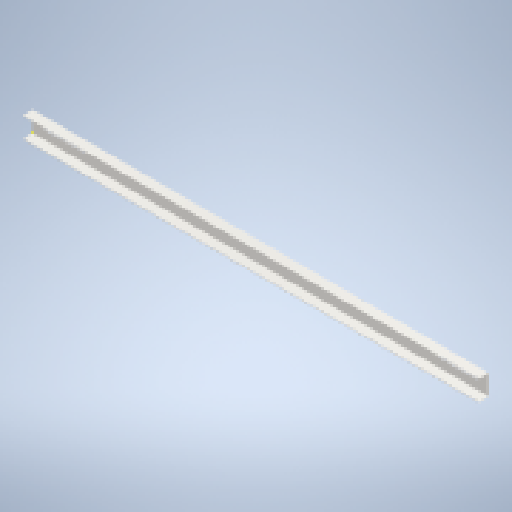
# Autodesk Inventor part: ThanhKe
Saved by Autodesk Inventor 2023 (Build 270158000, 158)
## iProperties
Created: 2025-03-24
Part Number: ThanhKe
Material: Generic
Document SubType Name: Modeling
Designer: huyqu
Density: 1 g/cm^3
Appearance: Default
Author: huyqu
Autodesk Inventor part; units mm, degrees
ref_plane "YZ Plane" through (0, 0, 0) normal (1, 0, 0) x (0, 1, 0)
ref_plane "XZ Plane" through (0, 0, 0) normal (0, 1, 0) x (-1, 0, 0)
ref_plane "XY Plane" through (0, 0, 0) normal (0, 0, 1) x (1, 0, 0)
sketch "Sketch1" plane through (0, 0, 0) normal (0, 0, 1) x (1, 0, 0)
  line L0 (0, 0) -> (2200, 0)
  line L1 (0, 0) -> (0, -3)
  line L2 (0, -3) -> (2200, -3)
  line L3 (2200, -3) -> (2200, 0)
  dimension "d0" = 2200
  dimension "d1" = 3
  dimension "d2" = 2200
  constraints: 8 end point, 2 horizontal, 1 vertical
  measures "d0" distance of L0.start L0.end
  measures "d1" distance of L0.start L1.end
  measures "d2" distance of L1.end L2.end
extrude "Extrusion1" add sketch "Sketch1" along normal blind 50
sketch "Sketch2" plane through (0, 0, 0) normal (0, 1, 0) x (1, 0, 0)
  line L0 (0, 0) -> (0, -50) projected
  line L1 (0, -3) -> (2200, -3)
  line L2 (2200, 0) -> (0, 0) projected
  line L3 (0, -3) -> (0, 0)
  line L4 (0, 0) -> (2200, 0)
  line L5 (2200, 0) -> (2200, -50) projected
  line L6 (2200, 0) -> (2200, -3)
  dimension "d5" = 2200
  dimension "d6" = 3
  constraints: 8 end point, 1 collinear, 1 parallel, 1 perpendicular, 1 point on line
  measures "d5" distance of L1.start L1.end
  measures "d6" distance between parallel lines of L2 L1
extrude "Extrusion2" add sketch "Sketch2" along normal blind 97
sketch "Sketch3" plane through (0, 0, 3) normal (0, 0, 1) x (1, 0, 0)
  line L0 (0, -3) -> (0, 97) projected
  line L1 (0, 94) -> (2200, 94)
  line L2 (0, 97) -> (2200, 97) projected
  line L3 (0, 94) -> (0, 97)
  line L4 (0, 97) -> (2200, 97)
  line L5 (2200, 97) -> (2200, 94)
  point P0 (0, 0)
  dimension "d9" = 3
  dimension "d10" = 2200
  constraints: 8 end point, 2 perpendicular, 1 point on line
  measures "d9" distance between parallel lines of L1 L2
  measures "d10" distance of L1.start L1.end
extrude "Extrusion3" add sketch "Sketch3" along normal blind 47
fillet "Fillet1" radius 3 4 edges at (1100, -3, 0) (1100, 97, 0) (1100, 0, 3) (1100, 94, 3)
sketch "Sketch4" plane through (0, 0, 0) normal (0, 0, -1) x (-1, 0, 0)
  line L0 (0, 0) -> (0, 94) projected
  line L1 (-55, 52) -> (-250, 52)
  line L2 (-255.2761, 47.6162) -> (-255.2761, 46.4034)
  line L3 (-250.626, 42.0196) -> (-54.5576, 42.0196)
  arc A0 (-250, 52) -> (-250, 42.0196) centre (-250.313, 47.0098) ccw
  arc A1 (-55.4424, 42.0196) -> (-55, 52) centre (-55, 47) ccw
  dimension "d16" = 10
  constraints: 8 point on circle, 6 end point, 2 centre point, 2 point on line, 1 horizontal, 1 vertical
  measures "d16" distance of L1.end L3.start
extrude "Extrusion4" cut sketch "Sketch4" against normal through all contours A1 L3 A0 L2 L1
sketch "Sketch5" plane through (0, 0, 0) normal (0, 0, -1) x (-1, 0, 0)
  line L0 (-2200, 3) -> (-2200, 91) projected
  line L1 (-2145, 42) -> (-1955, 42)
  line L2 (-1955, 52) -> (-2145, 52)
  arc A0 (-2145, 52) -> (-2145, 42) centre (-2145, 47) ccw
  arc A1 (-1955, 42) -> (-1955, 52) centre (-1955, 47) ccw
  point P0 (0, 0)
  constraints: 4 end point, 4 point on circle, 2 centre point, 2 horizontal, 1 tangent
extrude "Extrusion5" cut sketch "Sketch5" against normal blind 10
sketch "Sketch8" plane through (0, 0, 0) normal (0, 0, -1) x (-1, 0, 0)
  point P0 (0, 0)
body "Solid1"
